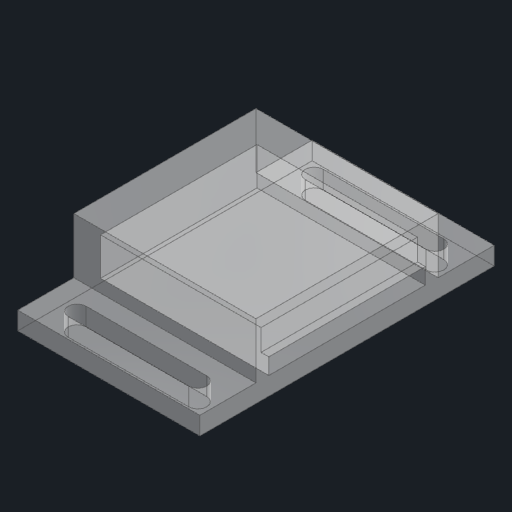
# Autodesk Inventor part: bottom
Saved by Autodesk Inventor 2023 (Build 270158030, 158C)
## iProperties
Created: 2022-07-13
Part Number: bottom
Material: SAN Plastic
Document SubType Name: Modeling
Designer: Norbert Ligas
Density: 1.068 g/cm^3
Appearance: Polycarbonate - Clear
width: 30,500 mm
length: 49,300 mm
opening_width: 3,000 mm
opening_length: 23,200 mm
opening_distance_to_edge: 3,300 mm
camera_box_width: 30,500 mm
thickness: 3,000 mm
inside_width: 26,200 mm
height: 12,300 mm
Author: Norbert Ligas
Autodesk Inventor part; units mm, degrees
ref_plane "YZ Plane" through (0, 0, 0) normal (1, 0, 0) x (0, 1, 0)
ref_plane "XZ Plane" through (0, 0, 0) normal (0, 1, 0) x (-1, 0, 0)
ref_plane "XY Plane" through (0, 0, 0) normal (0, 0, 1) x (1, 0, 0)
sketch "Sketch1" plane through (0, 0, 0) normal (0, 1, 0) x (-1, 0, 0)
  line L0 (15.25, -24.65) -> (-15.25, -24.65)
  line L1 (-15.25, -24.65) -> (-15.25, 24.65)
  line L2 (-15.25, 24.65) -> (15.25, 24.65)
  line L3 (15.25, 24.65) -> (15.25, -24.65)
  line L4 (15.25, -24.65) -> (-15.25, 24.65) construction
  line L5 (-15.25, -24.65) -> (15.25, 24.65) construction
  circle A0 centre (10.1, 19.85) radius 1.5
  circle A1 centre (-10.1, 19.85) radius 1.5
  line L6 (10.1, 21.35) -> (-10.1, 21.35)
  circle A2 centre (10.1, -19.85) radius 1.5
  circle A3 centre (-10.1, -19.85) radius 1.5
  line L7 (10.1, -21.35) -> (-10.1, -21.35)
  line L8 (21.35, 0) -> (-21.35, 0) construction
  line L9 (10.1, -18.35) -> (-10.1, -18.35)
  line L10 (10.1, 18.35) -> (-10.1, 18.35)
  line L11 (15.25, -15.25) -> (-15.25, -15.25)
  line L12 (-15.25, -15.25) -> (-15.25, 15.25)
  line L13 (-15.25, 15.25) -> (15.25, 15.25)
  line L14 (15.25, 15.25) -> (15.25, -15.25)
  line L15 (15.25, -15.25) -> (-15.25, 15.25) construction
  line L16 (-15.25, -15.25) -> (15.25, 15.25) construction
  line L17 (0, -34.51) -> (0, 34.51) projected
  point P0 (0, 0)
  dimension "d11" = 49.3
  dimension "d12" = 30.5
  dimension "d13" = 23.2
  dimension "d14" = 3
  dimension "d15" = 3.3
  dimension "d16" = 30.5
  constraints: 32 end point, 8 point on circle, 8 tangent, 6 parallel, 4 centre point, 4 midpoint, 2 horizontal, 2 perpendicular, 1 equal radius, 1 point on line, 1 symmetric about line, 4 other
  measures "d11" distance between parallel lines of L0 L2
  measures "d12" distance between parallel lines of L1 L3
  measures "d14" distance between parallel lines of L10 L6
  measures "d15" distance between parallel lines of L6 L2
  measures "d16" distance between parallel lines of L11 L13
extrude "Extrusion1" add sketch "Sketch1" along normal blind 3 contours L0 L17 L7 A2 L9 L11 L3 | L0 L1 L11 L17 L9 A3 L7 | L11 L17 L13 L3 | L13 L17 L10 A0 L6 L2 L3 | L11 L1 L13 L17 | L13 L1 L2 L17 L6 A1 L10
extrude "Extrusion2" add sketch "Sketch1" along normal blind 12.3 contours L11 L17 L13 L3 | L11 L1 L13 L17
sketch "Sketch2" plane through (0, 12.3, 0) normal (0, 1, 0) x (1, 0, 0)
  line L0 (12.9324, 13.1) -> (-12.9324, 13.1)
  line L1 (-12.9324, 13.1) -> (-12.9324, -13.1)
  line L2 (-12.9324, -13.1) -> (12.9324, -13.1)
  line L3 (12.9324, -13.1) -> (12.9324, 13.1)
  line L4 (12.9324, 13.1) -> (-12.9324, -13.1) construction
  line L5 (-12.9324, 13.1) -> (12.9324, -13.1) construction
  point P0 (0, 0)
  dimension "d21" = 26.2
  constraints: 12 end point, 2 midpoint, 2 parallel, 1 horizontal, 1 perpendicular
  measures "d21" distance between parallel lines of L0 L2
extrude "Extrusion3" cut sketch "Sketch2" against normal blind 9.3
sketch "Sketch3" plane through (12.9324, 12.3, -13.1) normal (-1, 0, 0) x (0, 0, 1)
  line L0 (26.2, 0) -> (26.2, -9.3) projected
  line L1 (26.2, -9.3) -> (0, -9.3) projected
  line L2 (0, 0) -> (0, -9.3) projected
  line L3 (-2.15, 0) -> (28.35, 0) projected
  line L4 (0, 0) -> (26.2, 0) projected
  line L5 (26.2, 0) -> (0, 0)
  line L6 (0, 0) -> (0, -9.3)
  line L7 (0, -9.3) -> (26.2, -9.3)
  line L8 (26.2, -9.3) -> (26.2, 0)
  point P0 (13.1, -12.3)
  constraints: 8 end point, 2 parallel, 1 horizontal, 1 perpendicular
extrude "Extrusion4" cut sketch "Sketch3" against normal through all
sketch "Sketch6" plane through (0, 12.3, 0) normal (0, 1, 0) x (1, 0, 0)
  line L0 (-15.25, 15.25) -> (-15.25, -15.25) projected
  line L1 (15.25, 15.25) -> (15.25, 24.65) projected
  line L2 (-15.25, -15.25) -> (15.25, -15.25)
  line L3 (15.25, -15.25) -> (15.25, 15.25)
  line L4 (15.25, 15.25) -> (-15.25, 15.25)
  line L5 (-15.25, 15.25) -> (-15.25, -15.25)
  point P0 (0, 0)
  constraints: 8 end point, 2 parallel, 1 horizontal, 1 perpendicular
extrude "Extrusion5" add sketch "Sketch6" against normal blind 3
sketch "Sketch7" plane through (0, 9.3, 0) normal (0, -1, 0) x (1, 0, 0)
  line L0 (15.25, 15.25) -> (15.25, -15.25) projected
  line L1 (-15.25, 15.25) -> (15.25, 15.25) projected
  line L2 (15.25, -15.25) -> (13.95, -15.25)
  line L3 (13.95, -15.25) -> (13.95, 15.25)
  line L4 (13.95, 15.25) -> (15.25, 15.25)
  line L5 (15.25, 15.25) -> (15.25, -15.25)
  line L6 (-15.25, -24.65) -> (-15.25, 24.65) projected
  point P0 (0, 0)
  dimension "d29" = 29.2
  constraints: 8 end point, 2 parallel, 1 horizontal, 1 perpendicular, 1 point on line
  measures "d29" distance between parallel lines of L3 L6
extrude "Extrusion6" add sketch "Sketch7" along normal blind 3.6
equation "\"d11\" = length"
equation "\"d12\" = width"
equation "\"d13\" = opening_length"
equation "\"d14\" = opening_width"
equation "\"d15\" = opening_distance_to_edge"
equation "\"d16\" = camera_box_width"
equation "\"d17\" = thickness"
equation "\"d19\" = height"
equation "\"d21\" = inside_width"
equation "\"d22\" = height - thickness"
equation "\"d26\" = thickness"
equation "\"d29\" = inside_width + thickness"
equation "\"d30\" = 1.2 * thickness"
equation "\"width\" = 30.5"
equation "\"length\" = 49.3"
equation "\"opening_width\" = 3"
equation "\"opening_length\" = 23.2"
equation "\"opening_distance_to_edge\" = 3.3"
equation "\"camera_box_width\" = 30.5"
equation "\"thickness\" = 3"
equation "\"inside_width\" = 26.2"
equation "\"height\" = 12.3"
body "Solid1"
